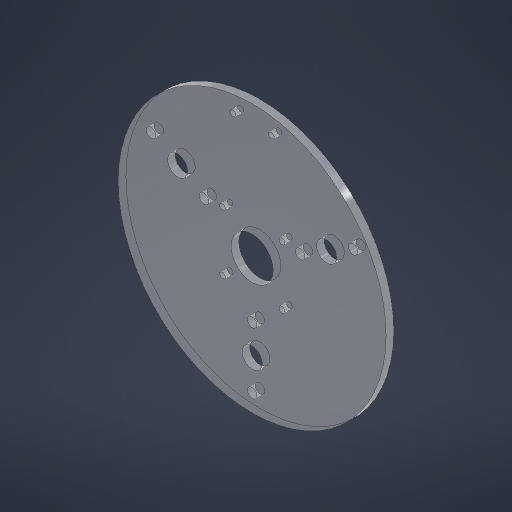
# Autodesk Inventor part: test_topo
Saved by Autodesk Inventor 2025.2 (Build 292293000, 293)
## iProperties
Created: 2025-05-02
Part Number: test_topo
Material: Generic
Document SubType Name: Modeling
Designer: Nelson
Density: 1 g/cm^3
Appearance: Polycarbonate - Clear
Author: Nelson
Autodesk Inventor part; units mm, degrees
ref_plane "YZ Plane" through (0, 0, 0) normal (1, 0, 0) x (0, 1, 0)
ref_plane "XZ Plane" through (0, 0, 0) normal (0, 1, 0) x (-1, 0, 0)
ref_plane "XY Plane" through (0, 0, 0) normal (0, 0, 1) x (1, 0, 0)
sketch "Sketch1" plane through (0, 0, 0) normal (0, 0, 1) x (1, 0, 0)
  circle A0 centre (0, 0) radius 70
  circle A1 centre (0, -45) radius 5.25
  circle A2 centre (0, 0) radius 11
  circle A3 centre (10.001, 60.58) radius 1.5
  circle A4 centre (-10.001, 60.58) radius 1.5
  circle A5 centre (15.4998, 15.4998) radius 1.5
  circle A6 centre (0, -29) radius 2.5
  circle A7 centre (0, -61) radius 2.5
  circle A8 centre (52.8275, 30.5) radius 2.5
  circle A9 centre (38.9711, 22.5) radius 5.25
  circle A10 centre (25.1147, 14.5) radius 2.5
  circle A11 centre (-52.8275, 30.5) radius 2.5
  circle A12 centre (-38.9711, 22.5) radius 5.25
  circle A13 centre (-25.1147, 14.5) radius 2.5
  circle A14 centre (0, 0) radius 21.92 construction
  circle A15 centre (-15.4998, 15.4998) radius 1.5
  circle A16 centre (-15.4998, -15.4998) radius 1.5
  circle A17 centre (15.4998, -15.4998) radius 1.5
  dimension "d53" = 43.84
  dimension "D_B" = 140
  dimension "Furos" = 10.5
  dimension "d11" = 22
  dimension "d24" = 3
  dimension "d25" = 3
  dimension "FN" = 3
  dimension "d31" = 5
  dimension "d32" = 5
  dimension "d34" = 16
  dimension "d35" = 16
  dimension "d36" = 10.001
  dimension "d37" = 10.001
  dimension "d38" = 60.58
  dimension "d39" = 60.58
  dimension "d40" = 45
  dimension "d50" = 360
  dimension "d56" = 360
  dimension "d58" = 15.4998
  dimension "d59" = 15.4998
  constraints: 17 centre point, 6 coincident, 4 vertical alignment, 31 other
  measures "D_B" diameter of A0
  measures "Furos" diameter of A1
  measures "d11" diameter of A2
  measures "d24" diameter of A3
  measures "d25" diameter of A4
  measures "FN" diameter of A5
  measures "d31" diameter of A6
  measures "d32" diameter of A7
  measures "d34" distance of A1.centre A6.centre
  measures "d35" distance of A7.centre A1.centre
  measures "d36" horizontal distance of A0.centre A4.centre
  measures "d37" horizontal distance of point (0, 0) A3.centre
  measures "d38" vertical distance of point (0, 0) A3.centre
  measures "d39" vertical distance of point (0, 0) A4.centre
  measures "d40" distance of point (0, 0) A1.centre
  measures "d58" horizontal distance of point (0, 0) A5.centre
  measures "d59" horizontal distance of point (0, 0) A5.centre
extrude "Extrusion1" add sketch "Sketch1" along normal blind 4
body "Solid1"
